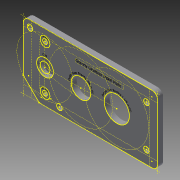
# Autodesk Inventor part: Granny Gearbox Input Plate
Saved by Autodesk Inventor 2015 (Build 190159000, 159)
## iProperties
Created: 2016-02-25
Part Number: Granny Gearbox Input Plate
Material: Generic
Document SubType Name: Modeling
Designer: sethbattis
Density: 1 g/cm^3
Appearance: Default
Author: sethbattis
Autodesk Inventor part; units mm, degrees
ref_plane "YZ Plane" through (0, 0, 0) normal (1, 0, 0) x (0, 1, 0)
ref_plane "XZ Plane" through (0, 0, 0) normal (0, 1, 0) x (-1, 0, 0)
ref_plane "XY Plane" through (0, 0, 0) normal (0, 0, 1) x (1, 0, 0)
derived "Granny Gearbox Output Plate.ipt"
sketch "Shaft Alignment" plane through (0, 0, 0) normal (0, 0, 1) x (1, 0, 0)
  circle A0 centre (40.6908, 0) radius 14.2875
  circle A1 centre (0, 0) radius 11.1125
  circle A2 centre (-40.7035, -0.0359) radius 5.5626
  line L0 (11.1125, 0) -> (11.1125, 11.8355) construction
  line L1 (26.4033, 0) -> (26.4033, 12.8304) construction
  circle A3 centre (-40.7035, 25.3641) radius 5.5626
  circle A4 centre (-40.7035, -25.4359) radius 5.5626
  line L2 (-40.7035, -0.0359) -> (0, 0) construction
  line L3 (0, 0) -> (40.6908, 0) construction
  line L4 (-40.7035, 25.3641) -> (-40.7035, -25.4359) construction
  line L5 (-46.2661, 25.3641) -> (-46.2661, -25.4359) construction
  line L6 (-40.7035, -5.5985) -> (-46.2661, -5.5985) construction
  line L7 (-40.7035, -19.8733) -> (-46.2661, -19.8733) construction
  line L8 (-40.7035, 19.8015) -> (-46.2661, 19.8015) construction
  line L9 (-40.7035, 5.5267) -> (-46.2661, 5.5267) construction
  line L10 (-40.7035, -5.5985) -> (-0.0001, -11.1125) construction
  line L11 (-35.1409, -0.031) -> (-35.1353, -6.3528) construction
  line L12 (-11.1125, -0.0098) -> (-11.104, -9.6083) construction
  line L13 (0, 11.1125) -> (43.74, 13.9583) construction
  point P0 (-33.5787, -27.5177)
sketch "New Mounting Holes" plane through (0, 0, 0) normal (0, 0, 1) x (1, 0, 0)
  circle A0 centre (74.3367, 23.3553) radius 3.175
  circle A1 centre (74.3367, -23.3553) radius 3.175
  circle A2 centre (-57.7242, 30.4609) radius 3.175
  circle A3 centre (-24.3812, -30.912) radius 3.175
  line L0 (-65.3633, -38.1) -> (-65.3633, 38.1) construction
  line L1 (87.0367, -38.1) -> (-65.3633, -38.1) construction
  line L2 (87.0367, 38.1) -> (87.0367, -38.1) construction
  line L3 (-65.3633, 38.1) -> (87.0367, 38.1) construction
  line L4 (-55.8383, 38.1) -> (-55.8383, -38.1) construction
  line L5 (-65.3633, 28.575) -> (87.0367, 28.575) construction
  line L6 (-65.3633, -28.575) -> (87.0367, -28.575) construction
  line L7 (77.5117, 38.1) -> (77.5117, -38.1) construction
  circle A4 centre (-40.7035, -0.0359) radius 31.75 construction
  circle A5 centre (40.6908, 0) radius 36.195 construction
  circle A6 centre (0, 0) radius 36.195 construction
  line L8 (-57.7242, 30.4609) -> (-55.8383, 30.4609) construction
  line L9 (-57.7242, 30.4609) -> (-57.7242, 28.575) construction
sketch "Labels" plane through (0, 0, 0) normal (0, 0, 1) x (1, 0, 0)
  circle A0 centre (-40.7035, -0.0359) radius 5.5626
  circle A1 centre (-40.7035, 25.3641) radius 5.5626
  circle A2 centre (-40.7035, -25.4359) radius 5.5626
  circle A3 centre (0, 0) radius 11.1125
  circle A4 centre (40.6908, 0) radius 14.2875
  line L0 (-5.8677, 26.2224) -> (48.5566, 26.2224) construction
  line L1 (48.5566, 26.2224) -> (48.5566, 22.1963) construction
  line L2 (48.5566, 22.1963) -> (-5.8677, 22.1963) construction
  line L3 (-5.8677, 22.1963) -> (-5.8677, 26.2224) construction
sketch "Exterior" plane through (0, 0, 0) normal (0, 0, 1) x (1, 0, 0)
  line L0 (-59.0133, 38.1) -> (80.6867, 38.1)
  line L1 (87.0367, 31.75) -> (87.0367, -31.75)
  line L2 (80.6867, -38.1) -> (-44.6678, -38.1)
  arc A0 (87.0367, 31.75) -> (80.6867, 38.1) centre (80.6867, 31.75) ccw
  arc A1 (80.6867, -38.1) -> (87.0367, -31.75) centre (80.6867, -31.75) ccw
  arc A2 (-59.0133, 38.1) -> (-65.3633, 31.75) centre (-59.0133, 31.75) ccw
  circle A3 centre (-40.7035, -0.0359) radius 31.75 construction
  line L3 (-65.3633, -17.4045) -> (-65.3633, 31.75)
  line L4 (-63.5034, -21.8946) -> (-49.1579, -36.2401)
  line L5 (-65.3633, -38.1) -> (-65.3633, 38.1) construction
  line L6 (87.0367, -38.1) -> (-65.3633, -38.1) construction
  arc A4 (-49.1579, -36.2401) -> (-44.6678, -38.1) centre (-44.6678, -31.75) ccw
  arc A5 (-65.3633, -17.4045) -> (-63.5034, -21.8946) centre (-59.0133, -17.4045) ccw
  point P0 (87.0367, 38.1)
  point P1 (-65.3633, -20.0348)
  point P2 (-47.2981, -38.1)
sketch "Input Plate" plane through (0, 0, 0) normal (0, 0, 1) x (1, 0, 0)
  circle A0 centre (40.6908, 0) radius 14.2875 projected
  circle A1 centre (0, 0) radius 11.1125 projected
  circle A2 centre (-40.7035, 25.3641) radius 5.5626 projected
  circle A3 centre (-57.7242, 30.4609) radius 3.175 projected
  circle A4 centre (-40.7035, -25.4359) radius 5.5626 projected
  circle A5 centre (-24.3812, -30.912) radius 3.175 projected
  circle A6 centre (74.3367, 23.3553) radius 3.175 projected
  circle A7 centre (-40.7035, -0.0359) radius 5.5626
  circle A8 centre (0, 0) radius 11.1125
  circle A9 centre (40.6908, 0) radius 14.2875
  circle A10 centre (74.3367, 23.3553) radius 3.175
  circle A11 centre (-57.7242, 30.4609) radius 3.175
  circle A12 centre (-24.3812, -30.912) radius 3.175
  circle A13 centre (-40.7035, -0.0359) radius 9.525
  circle A14 centre (-40.7035, 25.3641) radius 2.667
  circle A15 centre (-40.7035, -25.4359) radius 2.667
  circle A16 centre (74.3367, -23.3553) radius 3.175 projected
  circle A17 centre (74.3367, -23.3553) radius 3.175
  line L0 (-65.3633, -38.1) -> (-65.3633, 38.1) construction
  line L1 (-59.0133, 38.1) -> (80.6867, 38.1)
  line L2 (87.0367, 31.75) -> (87.0367, -31.75)
  line L3 (80.6867, -38.1) -> (-44.8133, -38.1)
  line L4 (-63.5034, -22.0402) -> (-49.3035, -36.2401)
  line L5 (-65.3633, -17.55) -> (-65.3633, 31.75)
  arc A18 (-59.0133, 38.1) -> (-65.3633, 31.75) centre (-59.0133, 31.75) ccw
  arc A19 (87.0367, 31.75) -> (80.6867, 38.1) centre (80.6867, 31.75) ccw
  arc A20 (80.6867, -38.1) -> (87.0367, -31.75) centre (80.6867, -31.75) ccw
  arc A21 (-49.3035, -36.2401) -> (-44.8133, -38.1) centre (-44.8133, -31.75) ccw
  arc A22 (-65.3633, -17.55) -> (-63.5034, -22.0402) centre (-59.0133, -17.55) ccw
  point P0 (-59.0133, 38.1)
  point P1 (-65.3633, 31.75)
  point P2 (-65.3633, -17.7835)
  point P3 (87.0367, -38.1)
  point P4 (87.0367, 38.1)
  dimension "d1" = 19.05
  dimension "d2" = 5.334
  dimension "d5" = 6.35
  constraints: 15 centre point, 11 equal radius, 10 coincident, 10 end point, 10 point on circle, 10 tangent, 4 point on line, 2 parallel, 1 horizontal, 1 perpendicular
  measures "d1" diameter of A13
  measures "d2" diameter of A14
  measures "d5" radius of A18
extrude "Extrusion1" add sketch "Input Plate" against normal blind 6.35 contours A2 | A4 | L1 A19 L2 A20 L3 A21 L4 A22 L5 A18
sketch "Input Labels" plane through (0, 0, 0) normal (0, 0, 1) x (1, 0, 0)
  circle A0 centre (-40.7035, 25.3641) radius 2.667 projected
  circle A1 centre (-40.7035, -0.0359) radius 9.525 projected
  circle A2 centre (-40.7035, -25.4359) radius 2.667 projected
  circle A3 centre (0, 0) radius 11.1125 projected
  line L0 (-5.8677, 22.1963) -> (-5.8677, 26.2224) construction
  line L1 (-5.8677, 26.2224) -> (48.5566, 26.2224) construction
  line L2 (48.5566, 26.2224) -> (48.5566, 22.1963) construction
  line L3 (48.5566, 22.1963) -> (-5.8677, 22.1963) construction
  circle A4 centre (40.6908, 0) radius 14.2875 projected
  line L4 (-5.8677, 26.2224) -> (45.7507, 26.2224) construction
  line L5 (45.7507, 26.2224) -> (45.7507, 22.1963) construction
  line L6 (45.7507, 22.1963) -> (-5.8677, 22.1963) construction
  line L7 (-5.8677, 22.1963) -> (-5.8677, 26.2224) construction
  constraints: 2 collinear, 7 other
body "Solid1"
